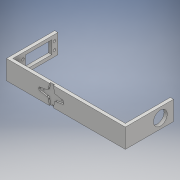
# Autodesk Inventor part: outerGantry
Saved by Autodesk Inventor 2018 (Build 220112000, 112)
## iProperties
Created: 2017-07-30
Part Number: outerGantry
Material: Generic
Document SubType Name: Modeling
Designer: kurtis
Density: 1 g/cm^3
Appearance: Default
Author: kurtis
Autodesk Inventor part; units mm, degrees
ref_plane "YZ Plane" through (0, 0, 0) normal (1, 0, 0) x (0, 1, 0)
ref_plane "XZ Plane" through (0, 0, 0) normal (0, 1, 0) x (-1, 0, 0)
ref_plane "XY Plane" through (0, 0, 0) normal (0, 0, 1) x (1, 0, 0)
sketch "Sketch1" plane through (0, 0, 0) normal (0, 0, 1) x (1, 0, 0)
  line L0 (0, 0) -> (175, 0)
  line L1 (0, 0) -> (0, 70)
  line L2 (0, 70) -> (-5, 70)
  line L3 (-5, 70) -> (-5, -5)
  line L4 (-5, -5) -> (180, -5)
  line L5 (180, -5) -> (180, 70)
  line L6 (180, 70) -> (175, 70)
  line L7 (175, 70) -> (175, 0)
  dimension "d0" = 175
  dimension "d1" = 70
  dimension "d2" = 5
  dimension "d3" = 75
  dimension "d4" = 185
  dimension "d5" = 75
  dimension "d6" = 5
  constraints: 16 end point, 3 vertical, 2 horizontal, 2 perpendicular
  measures "d0" distance of L0.start L0.end
  measures "d1" distance of L0.start L1.end
  measures "d2" distance of L1.end L2.end
  measures "d3" distance of L2.end L3.end
  measures "d4" distance of L3.end L4.end
  measures "d5" distance of L4.end L5.end
  measures "d6" distance of L5.end L6.end
extrude "Extrusion1" add sketch "Sketch1" along normal blind 30
sketch "Sketch2" plane through (-5, -5, 0) normal (-1, 0, 0) x (0, 0, 1)
  line L0 (0, 75) -> (30, 75) construction
  line L1 (15, 75) -> (15, 45) construction
  line L2 (5, 24.5) -> (25, 24.5)
  line L3 (25, 24.5) -> (25, 65.5)
  line L4 (25, 65.5) -> (5, 65.5)
  line L5 (5, 65.5) -> (5, 24.5)
  line L6 (5, 24.5) -> (25, 65.5) construction
  line L7 (25, 24.5) -> (5, 65.5) construction
  line L8 (5, 65.5) -> (5, 69.5) construction
  line L9 (5, 69.5) -> (9, 69.5) construction
  line L10 (25, 65.5) -> (25, 69.5) construction
  line L11 (25, 69.5) -> (21, 69.5) construction
  line L12 (5, 24.5) -> (5, 20.5) construction
  line L13 (5, 20.5) -> (9, 20.5) construction
  line L14 (25, 24.5) -> (25, 20.5) construction
  line L15 (25, 20.5) -> (21, 20.5) construction
  circle A0 centre (9, 69.5) radius 2
  circle A1 centre (21, 69.5) radius 2
  circle A2 centre (9, 20.5) radius 2
  circle A3 centre (21, 20.5) radius 2
  point P0 (0, 5)
  dimension "d9" = 30
  dimension "d10" = 20
  dimension "d11" = 41
  dimension "d12" = 4
  dimension "d13" = 4
  dimension "d14" = 4
  dimension "d15" = 4
  dimension "d16" = 4
  dimension "d17" = 4
  dimension "d18" = 4
  dimension "d19" = 4
  dimension "d20" = 4
  dimension "d21" = 4
  dimension "d22" = 4
  dimension "d23" = 4
  constraints: 30 end point, 5 perpendicular, 5 vertical, 4 centre point, 4 coincident, 3 midpoint, 2 parallel, 1 horizontal
  measures "d9" distance of L1.start L1.end
  measures "d10" distance of L4.end L3.end
  measures "d11" distance of L3.end L2.end
  measures "d12" distance of L4.end L8.end
  measures "d13" distance of L8.end L9.end
  measures "d14" distance of L3.end L10.end
  measures "d15" distance of L10.end L11.end
  measures "d16" distance of L2.start L12.end
  measures "d17" distance of L12.end L13.end
  measures "d18" distance of L2.end L14.end
  measures "d19" distance of L14.end L15.end
  measures "d20" diameter of A0
  measures "d21" diameter of A1
  measures "d22" diameter of A2
  measures "d23" diameter of A3
extrude "Extrusion2" cut sketch "Sketch2" against normal blind 10
sketch "Sketch3" plane through (175, 0, 0) normal (-1, 0, 0) x (0, 0, 1)
  line L0 (5, 60.5) -> (25, 60.5) construction
  line L1 (15, 60.5) -> (15, 49.5) construction
  circle A0 centre (15, 49.5) radius 10.75
  point P0 (0, 0)
  dimension "d26" = 11
  dimension "d27" = 21.5
  constraints: 2 end point, 1 centre point, 1 coincident, 1 midpoint, 1 vertical
  measures "d26" distance of L1.start L1.end
  measures "d27" diameter of A0
extrude "Extrusion3" cut sketch "Sketch3" against normal blind 14.5
sketch "Sketch4" plane through (-5, -5, 0) normal (0, -1, 0) x (1, 0, 0)
  line L0 (0, 25) -> (0, 5) construction
  line L1 (89.5, 14.2941) -> (89.5, 15.7059)
  line L2 (50.5, 15.7059) -> (50.5, 14.2941)
  line L3 (69.2941, 34.5) -> (70.7059, 34.5)
  line L4 (70.7059, -4.5) -> (69.2941, -4.5)
  line L5 (74.5, 22.5) -> (74.5, 21.5)
  line L6 (74.5, 8.5) -> (74.5, 7.5)
  line L7 (65.5, 7.5) -> (65.5, 8.5)
  line L8 (65.5, 21.5) -> (65.5, 22.5)
  line L9 (62.5, 10.5) -> (63.5, 10.5)
  line L10 (76.5, 10.5) -> (77.5, 10.5)
  line L11 (77.5, 19.5) -> (76.5, 19.5)
  line L12 (63.5, 19.5) -> (62.5, 19.5)
  arc A0 (63.5, 19.5) -> (65.5, 21.5) centre (63.5, 21.5) ccw
  arc A1 (74.5, 21.5) -> (76.5, 19.5) centre (76.5, 21.5) ccw
  arc A2 (76.5, 10.5) -> (74.5, 8.5) centre (76.5, 8.5) ccw
  arc A3 (65.5, 8.5) -> (63.5, 10.5) centre (63.5, 8.5) ccw
  line L13 (74.5, 22.5) -> (72.6755, 32.8473)
  line L14 (65.5, 22.5) -> (67.3245, 32.8473)
  line L15 (77.5, 10.5) -> (87.8473, 12.3245)
  line L16 (77.5, 19.5) -> (87.8473, 17.6755)
  line L17 (62.5, 19.5) -> (52.1527, 17.6755)
  line L18 (62.5, 10.5) -> (52.1527, 12.3245)
  line L19 (65.5, 7.5) -> (67.3245, -2.8473)
  line L20 (74.5, 7.5) -> (72.6755, -2.8473)
  arc A4 (52.1527, 17.6755) -> (50.5, 15.7059) centre (52.5, 15.7059) ccw
  arc A5 (50.5, 14.2941) -> (52.1527, 12.3245) centre (52.5, 14.2941) ccw
  arc A6 (69.2941, 34.5) -> (67.3245, 32.8473) centre (69.2941, 32.5) ccw
  arc A7 (72.6755, 32.8473) -> (70.7059, 34.5) centre (70.7059, 32.5) ccw
  arc A8 (89.5, 15.7059) -> (87.8473, 17.6755) centre (87.5, 15.7059) ccw
  arc A9 (87.8473, 12.3245) -> (89.5, 14.2941) centre (87.5, 14.2941) ccw
  arc A10 (67.3245, -2.8473) -> (69.2941, -4.5) centre (69.2941, -2.5) ccw
  arc A11 (70.7059, -4.5) -> (72.6755, -2.8473) centre (70.7059, -2.5) ccw
  line L21 (70, 15) -> (56, 15) construction
  line L22 (70, 15) -> (70, 29) construction
  line L23 (70, 15) -> (84, 15) construction
  line L24 (70, 15) -> (70, 1) construction
  circle A12 centre (70, 29) radius 0.75
  circle A13 centre (56, 15) radius 0.75
  circle A14 centre (84, 15) radius 0.75
  circle A15 centre (70, 1) radius 0.75
  point P0 (5, 0)
  point P1 (70, 15)
  dimension "d35" = 2
  dimension "d37" = 10
  dimension "d39" = 10
  dimension "d41" = 10
  dimension "d43" = 10
  dimension "d45" = 10
  dimension "d47" = 10
  dimension "d49" = 10
  dimension "d51" = 10
  dimension "d52" = 2
  dimension "d53" = 2
  dimension "d54" = 70
  dimension "d55" = 6.5
  dimension "d56" = 6.5
  dimension "d57" = 14
  dimension "d58" = 14
  dimension "d59" = 14
  dimension "d60" = 14
  dimension "d61" = 1.5
  dimension "d62" = 1.5
  dimension "d63" = 1.5
  dimension "d64" = 1.5
  constraints: 48 end point, 28 tangent, 24 point on circle, 16 centre point, 10 parallel, 9 equal radius, 5 horizontal, 4 coincident, 4 perpendicular, 2 vertical
  measures "d35" radius of A0
  measures "d37" angle of L5 L13
  measures "d39" angle of L8 L14
  measures "d41" angle of L10 L15
  measures "d43" angle of L11 L16
  measures "d45" angle of L12 L17
  measures "d47" angle of L9 L18
  measures "d49" angle of L7 L19
  measures "d51" angle of L6 L20
  measures "d52" radius of A4
  measures "d53" radius of A6
  measures "d54" distance from line of point (70, 15) L0
  measures "d55" horizontal distance of point (70, 15) A0.centre
  measures "d56" horizontal distance of point (70, 15) A0.centre
  measures "d57" distance of L21.start L21.end
  measures "d58" distance of L21.start L22.end
  measures "d59" distance of L21.start L23.end
  measures "d60" distance of L21.start L24.end
  measures "d61" diameter of A12
  measures "d62" diameter of A13
  measures "d63" diameter of A14
  measures "d64" diameter of A15
extrude "Extrusion4" cut sketch "Sketch4" against normal blind 2
extrude "Extrusion5" cut sketch "Sketch4" against normal blind 22 contours A12 | A13 | A14 | A15
equation "\"d3\" = d1 + d2"
equation "\"d4\" = d0 + 2 * d2"
equation "\"d5\" = d3"
equation "\"d6\" = d2"
equation "\"d14\" = d12"
equation "\"d15\" = d13"
equation "\"d16\" = d12"
equation "\"d17\" = d13"
equation "\"d18\" = d12"
equation "\"d19\" = d13"
equation "\"d39\" = d37"
equation "\"d41\" = d37"
equation "\"d43\" = d37"
equation "\"d45\" = d37"
equation "\"d47\" = d37"
equation "\"d49\" = d37"
equation "\"d51\" = d37"
equation "\"d58\" = d57"
equation "\"d59\" = d57"
equation "\"d60\" = d57"
equation "\"d62\" = d61"
equation "\"d63\" = d61"
equation "\"d64\" = d61"
body "Solid1"
